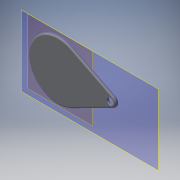
# Autodesk Inventor part: trapdoor_servo
Saved by Autodesk Inventor 2019 (Build 230136000, 136)
## iProperties
Created: 2019-01-09
Part Number: trapdoor_servo
Material: PET Plastic
Document SubType Name: Modeling
Designer: jmc
Density: 1.541 g/cm^3
Appearance: Polycarbonate - Clear
Author: jmc
Autodesk Inventor part; units mm, degrees
ref_plane "YZ Plane" through (0, 0, 0) normal (1, 0, 0) x (0, 1, 0)
ref_plane "XZ Plane" through (0, 0, 0) normal (0, 1, 0) x (-1, 0, 0)
ref_plane "XY Plane" through (0, 0, 0) normal (0, 0, 1) x (1, 0, 0)
ref_plane "Work Plane1" through (0, 0, 0) normal (0, 0, -1) x (-1, 0, 0)
ref_plane "Work Plane3" through (-59.1654, 22.8024, -1.2767) normal (0, 0, 1) x (0, 1, 0)
sketch "Sketch4" plane through (-59.1654, 22.8024, -1.2767) normal (0, 0, 1) x (0, 1, 0)
  line L0 (0, 0.2578) -> (0, -48.4285) construction
  line L1 (-4.3051, -44.7422) -> (4.9106, -44.7422) construction
  circle A0 centre (0, -44.7422) radius 2.97
  circle A1 centre (0, 0) radius 25.1499 construction
  arc A2 (-4.4358, -46.9838) -> (4.4358, -46.9838) centre (0, -44.7422) ccw
  line L2 (0, -55.7616) -> (-22.5832, -11.0728)
  line L3 (0, -55.7616) -> (22.4465, -11.3432)
  arc A3 (22.4465, -11.3432) -> (-22.4465, -11.3432) centre (0, 0) ccw
  line L4 (0, 0) -> (0, -25.1499) construction
  line L5 (0, -41.7722) -> (0, -73.1545) construction
  point P0 (-22.8024, -59.1654)
  dimension "d9" = 5.94
  dimension "d8" = 45
  dimension "d10" = 2
  constraints: 12 end point, 7 point on circle, 6 point on line, 3 centre point, 3 coincident, 3 vertical, 2 tangent, 1 concentric, 1 horizontal, 1 vertical alignment, 2 other
  measures "d8" distance from line of L0.start L1
extrude "Extrusion2" add sketch "Sketch4" along normal blind 2 contours L2 A3 L3 A2
fillet "Fillet2" radius 1.5 4 edges at (-9.4532, 22.8024, 0.7233) (-30.0019, 36.2436, 0.7233) (-84.3153, 22.8024, 0.7233) (-30.0019, 9.3612, 0.7233)
body "Solid2"
